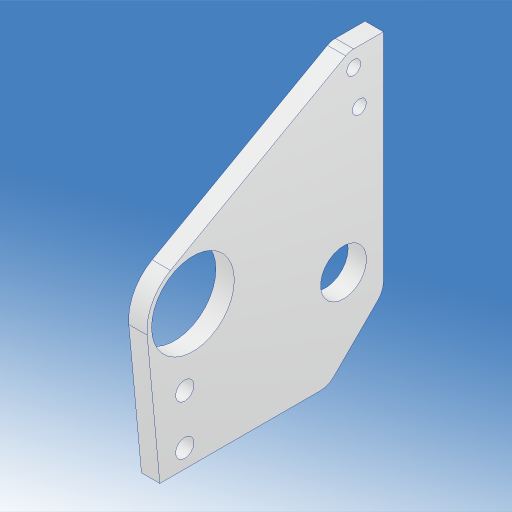
# Autodesk Inventor part: OuterDriveRail
Saved by Autodesk Inventor 2024 (Build 280153000, 153)
## iProperties
Created: 2023-02-06
Part Number: OuterDriveRail
Material: Aluminum 6061
Document SubType Name: Modeling
Designer: kumpu
Density: 2.7 g/cm^3
Appearance: Aluminum - Flat
Mass: 538.586 g
Surface Area: 696.12 cm^2
Volume: 199.476 cm^3
Author: kumpu
Autodesk Inventor part; units mm, degrees
ref_plane "YZ Plane" through (0, 0, 0) normal (1, 0, 0) x (0, 1, 0)
ref_plane "XZ Plane" through (0, 0, 0) normal (0, 1, 0) x (-1, 0, 0)
sketch "Sketch1" plane through (0, 0, 0) normal (1, 0, 0) x (0, 1, 0)
  line L0 (111.125, 190.5) -> (68.3957, 190.5)
  line L1 (20.2274, 160.5064) -> (-11.1661, 102.5705)
  arc A0 (-11.1661, 102.5705) -> (-11.1661, 90.4695) centre (0, 96.52) ccw
  line L2 (-11.1661, 90.4695) -> (7.6076, 55.8231)
  arc A1 (-11.1661, 6.0505) -> (-11.1661, -6.0505) centre (0, 0) ccw
  line L3 (-11.1661, -6.0505) -> (7.6076, -40.6969)
  arc A2 (-11.1661, -90.4695) -> (-11.3095, -102.2979) centre (0, -96.52) ccw
  line L4 (-11.3095, -102.2979) -> (18.6694, -160.9782)
  line L5 (67.5494, -190.5) -> (111.125, -190.5)
  line L6 (111.125, -190.5) -> (111.125, 190.5)
  arc A3 (20.2274, 160.5064) -> (68.3957, 190.5) centre (42.5128, 178.392) ccw
  arc A4 (67.5494, -190.5) -> (18.6694, -160.9782) centre (42.5128, -176.727) ccw
  circle A5 centre (42.5128, 178.392) radius 4.7625 construction
  circle A6 centre (34.925, -92.075) radius 7.9375 projected
  circle A7 centre (73.5908, -125.0234) radius 6.35 construction
  circle A8 centre (42.5128, -176.727) radius 4.7625 construction
  line L7 (111.125, 0) -> (0, 0) construction
  circle A9 centre (0, 96.52) radius 2.4892 construction
  circle A10 centre (0, 0) radius 2.4892 construction
  circle A11 centre (0, -96.52) radius 2.4892 construction
  line L8 (-11.1661, 6.0505) -> (7.6076, 40.6969)
  arc A12 (7.6076, 40.6969) -> (7.6076, 55.8231) centre (-6.35, 48.26) ccw
  line L9 (-11.1661, -90.4695) -> (7.6076, -55.8231)
  arc A13 (7.6076, -55.8231) -> (7.6076, -40.6969) centre (-6.35, -48.26) ccw
  line L10 (-6.35, -48.26) -> (-6.35, 48.26) construction
  line L11 (-6.35, 0) -> (0, 0) construction
  circle A14 centre (0, 96.52) radius 3.175
  circle A15 centre (0, 0) radius 3.175
  circle A16 centre (0, -96.52) radius 3.175
  circle A17 centre (46.0375, 122.682) radius 3.5687 construction
  circle A18 centre (20.6375, 122.682) radius 3.5687 construction
  circle A19 centre (46.0375, 122.682) radius 3.175
  circle A20 centre (20.6375, 122.682) radius 3.175
  line L12 (0, 96.52) -> (-12.7, 96.52) construction
  circle A21 centre (99.3625, 57.065) radius 2.0193
  circle A22 centre (47.625, -17.78) radius 2.0193
  circle A23 centre (99.3625, 31.665) radius 2.0193
  circle A24 centre (73.9625, 57.065) radius 2.0193
  circle A25 centre (73.9625, 31.665) radius 2.0193
  circle A26 centre (47.625, -43.18) radius 2.0193
  circle A27 centre (22.225, -17.78) radius 2.0193
  circle A28 centre (22.225, -43.18) radius 2.0193
  circle A29 centre (85.725, 107.103) radius 7.9375
  line L13 (-12.7, 173.6352) -> (-12.7, -210.2893) construction
  circle A30 centre (85.725, 107.103) radius 17.78 construction
  circle A31 centre (79.375, 147.2439) radius 22.86 construction
  circle A32 centre (42.5128, 178.392) radius 25.4 construction
  line L14 (110.475, 71.035) -> (60.975, 71.035) construction
  line L15 (60.975, 71.035) -> (60.975, -72.669) construction
  line L16 (60.975, -72.669) -> (110.475, -72.669) construction
  line L17 (110.475, -72.669) -> (110.475, 71.035) construction
  line L18 (58.7375, 86.554) -> (9.2375, 86.554) construction
  line L19 (9.2375, 86.554) -> (9.2375, -57.15) construction
  line L20 (9.2375, -57.15) -> (58.7375, -57.15) construction
  line L21 (58.7375, -57.15) -> (58.7375, 86.554) construction
  line L22 (9.525, 127) -> (-15.875, 127) construction
  line L23 (-15.875, 127) -> (-15.875, -177.8) construction
  line L24 (-15.875, -177.8) -> (9.525, -177.8) construction
  line L25 (9.525, -177.8) -> (9.525, 127) construction
  circle A33 centre (34.925, -92.075) radius 17.78 construction
  circle A34 centre (73.5908, -125.0234) radius 28.575 construction
  circle A35 centre (42.5128, -176.727) radius 31.75 construction
  circle A36 centre (102.0089, 180.2336) radius 2.413
  circle A37 centre (89.3089, 182.1987) radius 2.413
  circle A38 centre (102.0089, -180.2336) radius 2.413
  circle A39 centre (89.3089, -182.1987) radius 2.413
  circle A40 centre (79.375, 147.2439) radius 14.2875
  circle A41 centre (66.675, 254) radius 60.325 construction
  circle A42 centre (66.675, -254) radius 60.325 construction
  circle A43 centre (73.5908, -125.0234) radius 14.2875
  circle A44 centre (80.899, -155.6385) radius 47.527 construction
  circle A45 centre (100.0125, -85.369) radius 3.175
  circle A46 centre (74.6125, -85.369) radius 3.175
  circle A47 centre (100.0125, -85.369) radius 6.35 construction
  circle A48 centre (74.6125, -85.369) radius 6.35 construction
  circle A49 centre (46.0375, 122.682) radius 6.35 construction
  circle A50 centre (20.6375, 122.682) radius 6.35 construction
  circle A51 centre (34.6075, -121.8815) radius 3.175
  circle A52 centre (17.4625, -121.8815) radius 3.175
  circle A53 centre (34.6075, -121.8815) radius 6.35 construction
  circle A54 centre (17.4625, -121.8815) radius 6.35 construction
  circle A55 centre (101.6, 78.9725) radius 3.175
  circle A56 centre (101.6, 78.9725) radius 6.35 construction
  line L26 (92.075, 107.103) -> (79.375, 107.103) construction
  line L27 (79.375, 107.103) -> (79.375, 71.035) construction
  line L28 (79.375, 71.035) -> (92.075, 71.035) construction
  line L29 (92.075, 71.035) -> (92.075, 107.103) construction
  line L30 (85.725, 107.103) -> (85.725, 71.035) construction
  circle A57 centre (69.85, 78.9725) radius 3.175
  circle A58 centre (69.85, 78.9725) radius 6.35 construction
  circle A59 centre (59.143, -124.7108) radius 14.2875
  circle A60 centre (59.143, -124.7108) radius 22.86 construction
  dimension "d2" = 15.875
  dimension "d3" = 6.35
  dimension "d4" = 96.52
  dimension "d8" = 6.35
  dimension "d9" = 381
  dimension "d11" = 28.575
  dimension "d12" = 12.7
  dimension "d135" = 4.0386
  dimension "d136" = 4.0386
  dimension "d139" = 25.4
  dimension "d142" = 25.4
  dimension "d147" = 25.4
  dimension "d150" = 25.4
  dimension "d155" = 12.7
  dimension "d156" = 48.895
  dimension "d225" = 15.875
  dimension "d226" = 25.4
  dimension "d227" = 50.038
  dimension "d229" = 123.825
  dimension "d230" = 35.56
  dimension "d231" = 45.72
  dimension "d232" = 50.8
  dimension "d233" = 49.5
  dimension "d234" = 143.704
  dimension "d235" = 13.97
  dimension "d236" = 11.1125
  dimension "d237" = 143.704
  dimension "d238" = 49.5
  dimension "d239" = 11.1125
  dimension "d240" = 13.97
  dimension "d242" = 25.4
  dimension "d243" = 304.8
  dimension "d245" = 9.525
  dimension "d246" = 35.56
  dimension "d247" = 57.15
  dimension "d248" = 63.5
  dimension "d249" = 28.575
  dimension "d250" = 31.75
  dimension "d251" = 4.826
  dimension "d252" = 4.826
  dimension "d253" = 4.826
  dimension "d254" = 4.826
  dimension "d256" = 9.1161
  dimension "d257" = 12.7
  dimension "d258" = 1.9652
  dimension "d259" = 10.2664
  dimension "d260" = 12.7
  dimension "d261" = 1.9652
  dimension "d262" = 9.1161
  dimension "d263" = 10.2664
  dimension "d264" = 120.65
  dimension "d265" = 120.65
  dimension "d266" = 44.45
  dimension "d267" = 63.5
  dimension "d268" = 63.5
  dimension "d269" = 28.575
  dimension "d270" = 98.3615
  dimension "d271" = 14.224
  dimension "d272" = 95.054
  dimension "d273" = 6.35
  dimension "d274" = 6.35
  dimension "d275" = 25.4
  dimension "d276" = 11.1125
  dimension "d277" = 12.7
  constraints: 62 end point, 52 centre point, 25 coincident, 15 point on circle, 15 tangent, 10 equal radius, 10 horizontal, 8 parallel, 5 midpoint, 5 perpendicular, 5 vertical, 3 horizontal alignment, 2 concentric, 1 equal length, 1 vertical alignment, 13 other
  measures "d2" radius of A12
  measures "d3" distance from line of L7.end L10
  measures "d4" distance of L10.start L10.end
  measures "d8" diameter of A14
  measures "d9" distance of L5.end L0.start
  measures "d11" radius of A3
  measures "d12" radius of A0
  measures "d135" diameter of A21
  measures "d136" diameter of A22
  measures "d139" distance of A21.centre A23.centre
  measures "d142" distance of A21.centre A24.centre
  measures "d147" distance of A22.centre A26.centre
  measures "d150" distance of A22.centre A27.centre
  measures "d155" horizontal distance of A6.centre A28.centre
  measures "d156" vertical distance of A6.centre A28.centre
  measures "d225" diameter of A29
  measures "d226" distance from line of A29.centre L6
  measures "d227" vertical distance of A24.centre A29.centre
  measures "d229" distance between parallel lines of L13 L6
  measures "d230" diameter of A30
  measures "d231" diameter of A31
  measures "d232" diameter of A32
  measures "d233" distance of L15.end L16.end
  measures "d234" distance of L16.end L14.start
  measures "d235" distance from line of A21.centre L14
  measures "d236" distance from line of L17 A23.centre
  measures "d237" distance of L20.end L18.start
  measures "d238" distance of L18.start L18.end
  measures "d239" distance from line of L21 A26.centre
  measures "d240" distance from line of L20 A28.centre
  measures "d242" distance of L24.end L23.end
  measures "d243" distance of L22.end L23.end
  measures "d245" distance from line of A0.centre L25
  measures "d246" diameter of A33
  measures "d247" diameter of A34
  measures "d248" diameter of A35
  measures "d249" diameter of A40
  measures "d250" distance from line of A31.centre L6
  measures "d251" diameter of A36
  measures "d252" diameter of A37
  measures "d253" diameter of A38
  measures "d254" diameter of A39
  measures "d256" distance from line of A36.centre L6
  measures "d257" horizontal distance of A37.centre A36.centre
  measures "d258" vertical distance of A37.centre A36.centre
  measures "d259" distance from line of A36.centre L0
  measures "d260" horizontal distance of A39.centre A38.centre
  measures "d261" vertical distance of A39.centre A38.centre
  measures "d262" distance from line of L6 A38.centre
  measures "d263" distance from line of L5 A38.centre
  measures "d264" diameter of A41
  measures "d265" diameter of A42
  measures "d266" distance from line of A41.centre L6
  measures "d267" distance from line of L0 A41.centre
  measures "d268" distance from line of A42.centre L5
  measures "d269" diameter of A43
  measures "d270" vertical distance of A42.centre A44.centre
  measures "d271" horizontal distance of A42.centre A44.centre
  measures "d272" diameter of A44
  measures "d273" diameter of A46
  measures "d274" diameter of A45
  measures "d275" distance of A46.centre A45.centre
  measures "d276" distance from line of L6 A45.centre
  measures "d277" diameter of A48
ref_plane "Work Plane1" through (12.7, 0, 0) normal (1, 0, 0) x (0, 0, -1)
sketch "Sketch13" plane through (12.7, 0, 0) normal (1, 0, 0) x (0, 0, -1)
  circle A0 centre (180.2336, 102.0089) radius 2.413 projected
  circle A1 centre (182.1987, 89.3089) radius 2.413 projected
  circle A2 centre (176.727, 42.5128) radius 4.7625 construction
  line L0 (177.8, 9.525) -> (-127, 9.525) construction
  line L1 (177.8, -15.875) -> (177.8, 9.525) construction
  circle A3 centre (121.8815, 34.6075) radius 3.175 projected
  circle A4 centre (121.8815, 17.4625) radius 3.175 projected
  line L2 (190.5, 111.125) -> (-190.5, 111.125) projected
  line L3 (190.5, 72.4418) -> (190.5, 111.125) projected
  circle A5 centre (124.7108, 59.143) radius 15.875
  circle A6 centre (180.2336, 102.0089) radius 5.588
  circle A7 centre (182.1987, 89.3089) radius 5.588
  circle A8 centre (176.727, 42.5128) radius 7.9375
  circle A9 centre (121.8815, 34.6075) radius 6.35
  circle A10 centre (121.8815, 17.4625) radius 6.35
  circle A11 centre (125.0234, 73.5908) radius 28.575 construction
  circle A12 centre (92.075, 34.925) radius 22.225 construction
  circle A13 centre (176.727, 42.5128) radius 31.75 construction
  line L4 (116.9572, 72.9957) -> (177.5043, 106.8851)
  line L5 (180.2336, 107.5969) -> (190.5, 107.5969)
  line L6 (168.8197, 11.1125) -> (113.2813, 11.1125)
  line L7 (108.9055, 57.6571) -> (113.2813, 11.1125)
  line L8 (173.3099, 12.9724) -> (188.6401, 28.3026)
  line L9 (190.5, 72.4418) -> (190.5, 32.7928)
  arc A14 (168.8197, 11.1125) -> (173.3099, 12.9724) centre (168.8197, 17.4625) ccw
  arc A15 (188.6401, 28.3026) -> (190.5, 32.7928) centre (184.15, 32.7928) ccw
  circle A16 centre (124.7108, 59.143) radius 14.2875 projected
  point P0 (0, 0)
  point P1 (190.5, 30.1625)
  point P2 (171.45, 11.1125)
  point P3 (121.8815, 11.1125)
  dimension "d299" = 3.175
  dimension "d300" = 3.175
  dimension "d303" = 15.875
  dimension "d304" = 12.7
  dimension "d305" = 12.7
  dimension "d307" = 19.05
  dimension "d308" = 19.05
  dimension "d309" = 6.35
  dimension "d310" = 6.35
  dimension "d313" = 31.75
  constraints: 12 end point, 9 tangent, 8 centre point, 8 point on circle, 5 point on line, 4 coincident, 1 horizontal, 1 perpendicular, 1 vertical
  measures "d299" radial gap between concentric circles of A0 A6
  measures "d300" radial gap between concentric circles of A1 A7
  measures "d303" diameter of A8
  measures "d304" diameter of A9
  measures "d305" diameter of A10
  measures "d307" horizontal distance of point (190.5, 30.163) point (171.45, 11.113)
  measures "d308" horizontal distance of point (190.5, 30.163) point (171.45, 11.113)
  measures "d309" radius of A14
  measures "d310" radius of A15
  measures "d313" diameter of A5
extrude "Extrusion14" add sketch "Sketch13" along normal blind 6.35 contours A10 | L9 A15 L8 A14 L6 L7 A5 L4 A6 L5 L3 | A6 | A5 | A7 | A9
body "Solid2"
